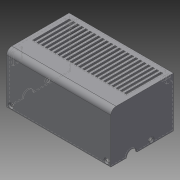
# Autodesk Inventor part: Top
Saved by Autodesk Inventor 2015 (Build 190159000, 159)
## iProperties
Created: 2019-01-20
Part Number: Top
Material: Generic
Document SubType Name: Modeling
Designer: Toby
Density: 1 g/cm^3
Appearance: Default
Author: Toby
Autodesk Inventor part; units mm, degrees
ref_plane "YZ Plane" through (0, 0, 0) normal (1, 0, 0) x (0, 1, 0)
ref_plane "XZ Plane" through (0, 0, 0) normal (0, 1, 0) x (-1, 0, 0)
ref_plane "XY Plane" through (0, 0, 0) normal (0, 0, 1) x (1, 0, 0)
sketch "Sketch1" plane through (0, 0, 0) normal (0, 0, 1) x (1, 0, 0)
  line L0 (-67.0623, 30.7122) -> (32.9377, 30.7122)
  line L1 (32.9377, 30.7122) -> (32.9377, -29.2878)
  line L2 (32.9377, -29.2878) -> (-67.0623, -29.2878)
  line L3 (-67.0623, -29.2878) -> (-67.0623, 30.7122)
  point P0 (0, 0)
  dimension "d0" = 100
  dimension "d1" = 60
  constraints: 8 end point, 2 parallel, 1 horizontal, 1 perpendicular
  measures "d0" distance of L0.start L0.end
  measures "d1" distance of L2.end L0.start
extrude "Extrusion1" add sketch "Sketch1" along normal blind 1.2
sketch "Sketch2" plane through (0, 0, 1.2) normal (0, 0, 1) x (1, 0, 0)
  line L0 (-67.0623, -29.2878) -> (32.9377, -29.2878) projected
  line L1 (-67.0623, 30.7122) -> (-65.8623, 30.7122)
  line L2 (-65.8623, 30.7122) -> (-65.8623, -29.2878)
  line L3 (-65.8623, -29.2878) -> (-67.0623, -29.2878)
  line L4 (-67.0623, -29.2878) -> (-67.0623, 30.7122)
  line L5 (32.9377, 30.7122) -> (31.7377, 30.7122)
  line L6 (31.7377, 30.7122) -> (31.7377, -29.2878)
  line L7 (31.7377, -29.2878) -> (32.9377, -29.2878)
  line L8 (32.9377, -29.2878) -> (32.9377, 30.7122)
  line L9 (31.7377, -29.2878) -> (-65.8623, -29.2878)
  line L10 (-65.8623, -29.2878) -> (-65.8623, -28.0878)
  line L11 (-65.8623, -28.0878) -> (31.7377, -28.0878)
  line L12 (31.7377, -28.0878) -> (31.7377, -29.2878)
  point P0 (0, 0)
  dimension "d4" = 1.2
  dimension "d5" = 1.2
  dimension "d6" = 1.2
  constraints: 24 end point, 6 parallel, 3 horizontal, 3 perpendicular, 3 point on line
  measures "d4" distance between parallel lines of L4 L2
  measures "d5" distance between parallel lines of L0 L11
  measures "d6" distance between parallel lines of L8 L6
extrude "Extrusion2" add sketch "Sketch2" against normal blind 48
fillet "Fillet1" radius 5 1 edges at (-17.0623, -29.2878, 1.2)
fillet "Fillet2" radius 5 1 edges at (-17.0623, -28.0878, 0)
sketch "Sketch3" plane through (0, 0, 1.2) normal (0, 0, 1) x (1, 0, 0)
  line L0 (32.9377, 30.7122) -> (-67.0623, 30.7122) projected
  line L1 (-67.0623, 30.7122) -> (-67.0623, -24.2878) projected
  line L2 (-62.0623, 25.7122) -> (-60.0623, 25.7122)
  line L3 (-60.0623, 25.7122) -> (-60.0623, -9.2878)
  line L4 (-60.0623, -9.2878) -> (-62.0623, -9.2878)
  line L5 (-62.0623, -9.2878) -> (-62.0623, 25.7122)
  line L6 (-56.0623, 25.7122) -> (-56.0623, -9.2878)
  line L7 (-56.0623, -9.2878) -> (-58.0623, -9.2878)
  line L8 (-58.0623, -9.2878) -> (-58.0623, 25.7122)
  line L9 (-52.0623, 25.7122) -> (-52.0623, -9.2878)
  line L10 (-52.0623, -9.2878) -> (-54.0623, -9.2878)
  line L11 (-54.0623, -9.2878) -> (-54.0623, 25.7122)
  line L12 (-48.0623, 25.7122) -> (-48.0623, -9.2878)
  line L13 (-48.0623, -9.2878) -> (-50.0623, -9.2878)
  line L14 (-50.0623, -9.2878) -> (-50.0623, 25.7122)
  line L15 (-46.0623, 25.7122) -> (-44.0623, 25.7122)
  line L16 (-44.0623, 25.7122) -> (-44.0623, -9.2878)
  line L17 (-44.0623, -9.2878) -> (-46.0623, -9.2878)
  line L18 (-46.0623, -9.2878) -> (-46.0623, 25.7122)
  line L19 (-42.0623, 25.7122) -> (-40.0623, 25.7122)
  line L20 (-40.0623, 25.7122) -> (-40.0623, -9.2878)
  line L21 (-40.0623, -9.2878) -> (-42.0623, -9.2878)
  line L22 (-42.0623, -9.2878) -> (-42.0623, 25.7122)
  line L23 (-38.0623, 25.7122) -> (-36.0623, 25.7122)
  line L24 (-36.0623, 25.7122) -> (-36.0623, -9.2878)
  line L25 (-36.0623, -9.2878) -> (-38.0623, -9.2878)
  line L26 (-38.0623, -9.2878) -> (-38.0623, 25.7122)
  line L27 (-34.0623, 25.7122) -> (-32.0623, 25.7122)
  line L28 (-32.0623, 25.7122) -> (-32.0623, -9.2878)
  line L29 (-32.0623, -9.2878) -> (-34.0623, -9.2878)
  line L30 (-34.0623, -9.2878) -> (-34.0623, 25.7122)
  line L31 (-30.0623, 25.7122) -> (-28.0623, 25.7122)
  line L32 (-28.0623, 25.7122) -> (-28.0623, -9.2878)
  line L33 (-28.0623, -9.2878) -> (-30.0623, -9.2878)
  line L34 (-30.0623, -9.2878) -> (-30.0623, 25.7122)
  line L35 (-26.0623, 25.7122) -> (-24.0623, 25.7122)
  line L36 (-24.0623, 25.7122) -> (-24.0623, -9.2878)
  line L37 (-24.0623, -9.2878) -> (-26.0623, -9.2878)
  line L38 (-26.0623, -9.2878) -> (-26.0623, 25.7122)
  line L39 (-22.0623, 25.7122) -> (-20.0623, 25.7122)
  line L40 (-20.0623, 25.7122) -> (-20.0623, -9.2878)
  line L41 (-20.0623, -9.2878) -> (-22.0623, -9.2878)
  line L42 (-22.0623, -9.2878) -> (-22.0623, 25.7122)
  line L43 (-18.0623, 25.7122) -> (-16.0623, 25.7122)
  line L44 (-16.0623, 25.7122) -> (-16.0623, -9.2878)
  line L45 (-16.0623, -9.2878) -> (-18.0623, -9.2878)
  line L46 (-18.0623, -9.2878) -> (-18.0623, 25.7122)
  line L47 (-14.0623, 25.7122) -> (-12.0623, 25.7122)
  line L48 (-12.0623, 25.7122) -> (-12.0623, -9.2878)
  line L49 (-12.0623, -9.2878) -> (-14.0623, -9.2878)
  line L50 (-14.0623, -9.2878) -> (-14.0623, 25.7122)
  line L51 (-10.0623, 25.7122) -> (-8.0623, 25.7122)
  line L52 (-8.0623, 25.7122) -> (-8.0623, -9.2878)
  line L53 (-8.0623, -9.2878) -> (-10.0623, -9.2878)
  line L54 (-10.0623, -9.2878) -> (-10.0623, 25.7122)
  line L55 (-6.0623, 25.7122) -> (-4.0623, 25.7122)
  line L56 (-4.0623, 25.7122) -> (-4.0623, -9.2878)
  line L57 (-4.0623, -9.2878) -> (-6.0623, -9.2878)
  line L58 (-6.0623, -9.2878) -> (-6.0623, 25.7122)
  line L59 (-2.0623, 25.7122) -> (-0.0623, 25.7122)
  line L60 (-0.0623, 25.7122) -> (-0.0623, -9.2878)
  line L61 (-0.0623, -9.2878) -> (-2.0623, -9.2878)
  line L62 (-2.0623, -9.2878) -> (-2.0623, 25.7122)
  line L63 (1.9377, 25.7122) -> (3.9377, 25.7122)
  line L64 (3.9377, 25.7122) -> (3.9377, -9.2878)
  line L65 (3.9377, -9.2878) -> (1.9377, -9.2878)
  line L66 (1.9377, -9.2878) -> (1.9377, 25.7122)
  line L67 (5.9377, 25.7122) -> (7.9377, 25.7122)
  line L68 (7.9377, 25.7122) -> (7.9377, -9.2878)
  line L69 (7.9377, -9.2878) -> (5.9377, -9.2878)
  line L70 (5.9377, -9.2878) -> (5.9377, 25.7122)
  line L71 (9.9377, 25.7122) -> (11.9377, 25.7122)
  line L72 (11.9377, 25.7122) -> (11.9377, -9.2878)
  line L73 (11.9377, -9.2878) -> (9.9377, -9.2878)
  line L74 (9.9377, -9.2878) -> (9.9377, 25.7122)
  line L75 (13.9377, 25.7122) -> (15.9377, 25.7122)
  line L76 (15.9377, 25.7122) -> (15.9377, -9.2878)
  line L77 (15.9377, -9.2878) -> (13.9377, -9.2878)
  line L78 (13.9377, -9.2878) -> (13.9377, 25.7122)
  line L79 (17.9377, 25.7122) -> (19.9377, 25.7122)
  line L80 (19.9377, 25.7122) -> (19.9377, -9.2878)
  line L81 (19.9377, -9.2878) -> (17.9377, -9.2878)
  line L82 (17.9377, -9.2878) -> (17.9377, 25.7122)
  line L83 (21.9377, 25.7122) -> (23.9377, 25.7122)
  line L84 (23.9377, 25.7122) -> (23.9377, -9.2878)
  line L85 (23.9377, -9.2878) -> (21.9377, -9.2878)
  line L86 (21.9377, -9.2878) -> (21.9377, 25.7122)
  line L87 (25.9377, 25.7122) -> (27.9377, 25.7122)
  line L88 (27.9377, 25.7122) -> (27.9377, -9.2878)
  line L89 (27.9377, -9.2878) -> (25.9377, -9.2878)
  line L90 (25.9377, -9.2878) -> (25.9377, 25.7122)
  point P0 (0, 0)
  point P1 (-64.0623, 25.7122)
  dimension "d11" = 5
  dimension "d12" = 5
  dimension "d13" = 2
  dimension "d14" = 35
  dimension "d15" = 2
  dimension "d16" = 2
  dimension "d17" = 2
  dimension "d18" = 35
  dimension "d19" = 2
  dimension "d20" = 2
  dimension "d21" = 35
  dimension "d22" = 2
  dimension "d23" = 2
  dimension "d24" = 35
  dimension "d25" = 2
  dimension "d26" = 35
  dimension "d27" = 2
  dimension "d28" = 35
  dimension "d29" = 2
  dimension "d30" = 35
  dimension "d31" = 2
  dimension "d32" = 35
  dimension "d33" = 2
  dimension "d34" = 35
  dimension "d35" = 2
  dimension "d36" = 35
  dimension "d37" = 2
  dimension "d38" = 35
  dimension "d39" = 2
  dimension "d40" = 35
  dimension "d41" = 2
  dimension "d42" = 35
  dimension "d43" = 2
  dimension "d44" = 35
  dimension "d45" = 2
  dimension "d46" = 35
  dimension "d47" = 2
  dimension "d48" = 35
  dimension "d49" = 2
  dimension "d50" = 35
  dimension "d51" = 2
  dimension "d52" = 35
  dimension "d53" = 2
  dimension "d54" = 35
  dimension "d55" = 2
  dimension "d56" = 35
  dimension "d57" = 2
  dimension "d58" = 35
  dimension "d59" = 2
  dimension "d60" = 35
  dimension "d61" = 2
  dimension "d62" = 35
  dimension "d63" = 2
  constraints: 178 end point, 43 parallel, 20 horizontal, 20 perpendicular
  measures "d11" distance from line of L0 L2.start
  measures "d12" distance from line of L1 L2.start
  measures "d13" distance of L2.start point (-60.062, 25.712)
  measures "d14" distance of L2.end L3.end
  measures "d15" distance between parallel lines of L5 L3
  measures "d16" distance from line of L5 point (-64.062, 25.712)
  measures "d17" distance of L8.end point (-56.062, 25.712)
  measures "d18" distance of L6.start L6.end
  measures "d19" distance between parallel lines of L8 L6
  measures "d20" distance of L11.end point (-52.062, 25.712)
  measures "d21" distance of L9.start L9.end
  measures "d22" distance between parallel lines of L11 L9
  measures "d23" distance of L14.end point (-48.062, 25.712)
  measures "d24" distance of L12.start L12.end
  measures "d25" distance between parallel lines of L14 L12
  measures "d26" distance of L15.end L16.end
  measures "d27" distance between parallel lines of L18 L16
  measures "d28" distance of L19.end L20.end
  measures "d29" distance between parallel lines of L22 L20
  measures "d30" distance of L23.end L24.end
  measures "d31" distance between parallel lines of L26 L24
  measures "d32" distance of L27.end L28.end
  measures "d33" distance between parallel lines of L30 L28
  measures "d34" distance of L31.end L32.end
  measures "d35" distance between parallel lines of L34 L32
  measures "d36" distance of L35.end L36.end
  measures "d37" distance between parallel lines of L38 L36
  measures "d38" distance of L39.end L40.end
  measures "d39" distance between parallel lines of L42 L40
  measures "d40" distance of L43.end L44.end
  measures "d41" distance between parallel lines of L46 L44
  measures "d42" distance of L47.end L48.end
  measures "d43" distance between parallel lines of L50 L48
  measures "d44" distance of L51.end L52.end
  measures "d45" distance between parallel lines of L54 L52
  measures "d46" distance of L55.end L56.end
  measures "d47" distance between parallel lines of L58 L56
  measures "d48" distance of L59.end L60.end
  measures "d49" distance between parallel lines of L62 L60
  measures "d50" distance of L63.end L64.end
  measures "d51" distance between parallel lines of L66 L64
  measures "d52" distance of L67.end L68.end
  measures "d53" distance between parallel lines of L70 L68
  measures "d54" distance of L71.end L72.end
  measures "d55" distance between parallel lines of L74 L72
  measures "d56" distance of L75.end L76.end
  measures "d57" distance between parallel lines of L78 L76
  measures "d58" distance of L79.end L80.end
  measures "d59" distance between parallel lines of L82 L80
  measures "d60" distance of L83.end L84.end
  measures "d61" distance between parallel lines of L86 L84
  measures "d62" distance of L87.end L88.end
  measures "d63" distance between parallel lines of L90 L88
extrude "Extrusion3" cut sketch "Sketch3" against normal blind 48
sketch "Sketch4" plane through (0, 0, 1.2) normal (0, 0, 1) x (1, 0, 0)
  line L0 (-58.0623, 25.7122) -> (-56.0623, 25.7122)
  line L1 (-56.0623, 25.7122) -> (-56.0623, -9.2878)
  line L2 (-56.0623, -9.2878) -> (-58.0623, -9.2878)
  line L3 (-58.0623, -9.2878) -> (-58.0623, 25.7122)
  line L4 (-62.0623, 25.7122) -> (-60.0623, 25.7122) projected
  line L5 (-60.0623, -9.2878) -> (-62.0623, -9.2878) projected
  line L6 (-60.0623, 25.7122) -> (-60.0623, -9.2878) projected
  line L7 (-54.0623, 25.7122) -> (-52.0623, 25.7122)
  line L8 (-52.0623, 25.7122) -> (-52.0623, -9.2878)
  line L9 (-52.0623, -9.2878) -> (-54.0623, -9.2878)
  line L10 (-54.0623, -9.2878) -> (-54.0623, 25.7122)
  line L11 (-50.0623, 25.7122) -> (-48.0623, 25.7122)
  line L12 (-48.0623, 25.7122) -> (-48.0623, -9.2878)
  line L13 (-48.0623, -9.2878) -> (-50.0623, -9.2878)
  line L14 (-50.0623, -9.2878) -> (-50.0623, 25.7122)
  point P0 (0, 0)
  dimension "d66" = 2
  dimension "d67" = 2
  dimension "d68" = 2
  dimension "d69" = 2
  constraints: 24 end point, 6 parallel, 3 horizontal, 3 perpendicular, 2 collinear, 1 coincident
  measures "d66" distance between parallel lines of L3 L1
  measures "d67" distance between parallel lines of L6 L3
  measures "d68" distance between parallel lines of L10 L8
  measures "d69" distance between parallel lines of L14 L12
extrude "Extrusion4" cut sketch "Sketch4" against normal blind 48
sketch "Sketch5" plane through (-67.0623, -29.2878, -46.8) normal (-1, 0, 0) x (0, 0, 1)
  line L0 (43, 14.5) -> (32, 14.5)
  line L1 (32, 14.5) -> (32, 5)
  line L2 (32, 5) -> (43, 5)
  line L3 (43, 5) -> (43, 14.5)
  line L4 (48, 60) -> (48, 5) projected
  line L5 (43, 0) -> (0, 0) projected
  point P0 (46.8, 29.2878)
  dimension "d72" = 11
  dimension "d73" = 9.5
  dimension "d74" = 5
  dimension "d75" = 5
  constraints: 8 end point, 2 parallel, 1 horizontal, 1 perpendicular
  measures "d72" distance of L0.start L0.end
  measures "d73" distance of L2.end L0.start
  measures "d74" distance between parallel lines of L4 L3
  measures "d75" distance between parallel lines of L5 L2
extrude "Extrusion5" cut sketch "Sketch5" against normal blind 48
sketch "Sketch6" plane through (-67.0623, -29.2878, -46.8) normal (0, -1, 0) x (1, 0, 0)
  line L0 (0, 43) -> (0, 0) projected
  line L1 (100, 0) -> (0, 0) projected
  line L2 (100, 43) -> (100, 0) projected
  point P0 (67.0623, 46.8)
  point P1 (4.2, 3)
  point P2 (95.8, 3)
  dimension "d78" = 4.2
  dimension "d79" = 3
  dimension "d80" = 3
  dimension "d81" = 4.2
  measures "d78" distance from line of L0 point (4.2, 3)
  measures "d79" distance from line of L1 point (4.2, 3)
  measures "d80" distance from line of L1 point (95.8, 3)
  measures "d81" distance from line of L2 point (95.8, 3)
hole "Hole1" at (-62.8623, -29.2878, -43.8) at (28.7377, -29.2878, -43.8) direction (0, 1, 0) diameter 3 depth 8 tip angle 118 countersink diameter 5 countersink angle 90
sketch "Sketch7" plane through (32.9377, -29.2878, -46.8) normal (1, 0, 0) x (0, 0, -1)
  line L0 (0, 60) -> (0, 0) projected
  line L1 (-43, 0) -> (0, 0) projected
  point P0 (-46.8, 29.2878)
  point P1 (-3, 39)
  dimension "d89" = 3
  dimension "d90" = 39
  measures "d89" distance from line of L0 point (-3, 39)
  measures "d90" distance from line of L1 point (-3, 39)
hole "Hole2" at (32.9377, 9.7122, -43.8) direction (-1, 0, 0) diameter 3 depth 8 tip angle 118 countersink diameter 5 countersink angle 90
sketch "Sketch8" plane through (-67.0623, -29.2878, -46.8) normal (-1, 0, 0) x (0, 0, 1)
  circle A0 centre (3, 39) radius 1.5 projected
  point P0 (46.8, 29.2878)
  constraints: 1 coincident
hole "Hole3" at (-67.0623, 9.7122, -43.8) direction (1, 0, 0) diameter 3 depth 8 tip angle 118 countersink diameter 5 countersink angle 90
sketch "Sketch9" plane through (-67.0623, 30.7122, 1.2) normal (0, 1, 0) x (1, 0, 0)
  line L0 (98.8, 1.2) -> (92.8, 1.2)
  line L1 (92.8, 1.2) -> (92.8, 7.2)
  line L2 (92.8, 7.2) -> (98.8, 7.2)
  line L3 (98.8, 7.2) -> (98.8, 1.2)
  line L4 (1.2, 1.2) -> (7.2, 1.2)
  line L5 (7.2, 1.2) -> (7.2, 7.2)
  line L6 (7.2, 7.2) -> (1.2, 7.2)
  line L7 (1.2, 7.2) -> (1.2, 1.2)
  point P0 (67.0623, 1.2)
  dimension "d105" = 6
  dimension "d106" = 6
  dimension "d107" = 6
  dimension "d108" = 6
  constraints: 16 end point, 4 parallel, 2 horizontal, 2 perpendicular
  measures "d105" distance of L1.end L2.end
  measures "d106" distance of L0.end L1.end
  measures "d107" distance of L6.end L5.end
  measures "d108" distance of L5.end L4.end
extrude "Extrusion6" add sketch "Sketch9" against normal blind 5
sketch "Sketch10" plane through (-67.0623, 30.7122, 1.2) normal (0, 1, 0) x (1, 0, 0)
  line L0 (7.2, 1.2) -> (7.2, 7.2) projected
  line L1 (7.2, 7.2) -> (1.2, 7.2) projected
  line L2 (92.8, 7.2) -> (98.8, 7.2) projected
  line L3 (92.8, 1.2) -> (92.8, 7.2) projected
  point P0 (67.0623, 1.2)
  point P1 (95.8, 4.2)
  point P2 (4.2, 4.2)
  dimension "d111" = 3
  dimension "d112" = 3
  dimension "d113" = 3
  dimension "d114" = 3
  measures "d111" distance from line of L0 point (4.2, 4.2)
  measures "d112" distance from line of L1 point (4.2, 4.2)
  measures "d113" distance from line of L2 point (95.8, 4.2)
  measures "d114" distance from line of L3 point (95.8, 4.2)
hole "Hole4" at (28.7377, 30.7122, -3) at (-62.8623, 30.7122, -3) direction (0, -1, 0) diameter 3 depth 8 tip angle 118
sketch "Sketch11" plane through (-67.0623, -29.2878, -46.8) normal (-1, 0, 0) x (0, 0, 1)
  line L0 (0, 60) -> (0, 1.2) projected
  line L1 (43, 0) -> (0, 0) projected
  circle A0 centre (0, 20) radius 5
  point P0 (46.8, 29.2878)
  dimension "d122" = 20
  dimension "d123" = 10
  constraints: 1 centre point, 1 coincident, 1 point on line
  measures "d122" distance from line of L1 point (0, 20)
  measures "d123" diameter of A0
extrude "Extrusion7" cut sketch "Sketch11" against normal blind 500
body "Solid1"
